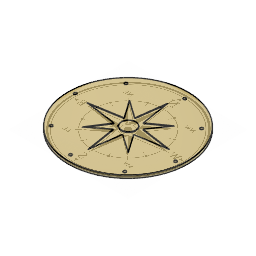
middle lid (Autodesk Fusion 360 design; units mm, degrees)
part number: 2026-06-30-11-55-46-724
Autodesk Fusion 360 part; units mm, degrees
sketch "Sketch1" plane through (0, 0, 0) normal (0, 1, 0) x (1, 0, 0)
  circle A0 centre (0, 0) radius 51
  dimension "d4" = 102
  constraint coincident A0.centre origin
  measures "d4" diameter of A0
sketch "Sketch2" plane through (0, 0, 0) normal (0, 1, 0) x (1, 0, 0)
  circle A0 centre (3.734, 44.6441) radius 1.2
  circle A1 centre (33.0064, 29.8467) radius 1.2
  circle A2 centre (46.1628, -5.5898) radius 1.2
  circle A3 centre (31.9934, -34.8384) radius 1.2
  circle A4 centre (-3.5224, -45.5641) radius 1.2
  circle A5 centre (-33.23, -32.3841) radius 1.2
  circle A6 centre (-46.7, 1.7546) radius 1.2
  circle A7 centre (-32.6391, 30.8334) radius 1.2
  dimension "d2" = 2.4
  dimension "d3" = 44.8
  dimension "d5" = 2.4
  dimension "d6" = 44.5
  dimension "d7" = 32.8
  dimension "d8" = 2.4
  dimension "d9" = 46.5
  dimension "d11" = 37.8
  dimension "d12" = 2.4
  dimension "d13" = 47.3
  dimension "d14" = 32.5
  dimension "d15" = 2.4
  dimension "d16" = 45.7
  dimension "d17" = 37.1
  dimension "d18" = 2.4
  dimension "d19" = 46.4
  dimension "d20" = 32.5
  dimension "d21" = 2.4
  dimension "d22" = 46.7
  dimension "d23" = 36.7
  dimension "d24" = 2.4
  dimension "d25" = 44.9
  dimension "d26" = 32.3
  dimension "d27" = 38.9067
  measures "d2" diameter of A0
  measures "d3" distance of A0.centre origin
  measures "d5" diameter of A1
  measures "d6" distance of origin A1.centre
  measures "d7" distance of A0.centre A1.centre
  measures "d8" diameter of A2
  measures "d9" distance of origin A2.centre
  measures "d11" distance of A1.centre A2.centre
  measures "d12" diameter of A3
  measures "d13" distance of origin A3.centre
  measures "d14" distance of A2.centre A3.centre
  measures "d15" diameter of A4
  measures "d16" distance of origin A4.centre
  measures "d17" distance of A3.centre A4.centre
  measures "d18" diameter of A5
  measures "d19" distance of origin A5.centre
  measures "d20" distance of A4.centre A5.centre
  measures "d21" diameter of A6
  measures "d22" horizontal distance of origin A6.centre
  measures "d23" distance of A5.centre A6.centre
  measures "d24" diameter of A7
  measures "d25" distance of origin A7.centre
  measures "d26" distance of A6.centre A7.centre
  measures "d27" distance of A0.centre A7.centre
extrude "Extrude1" add sketch "Sketch1" along normal blind 1.5
extrude "Extrude2" cut sketch "Sketch2" along normal blind 1.5
sketch "Sketch3" plane through (0, 0, 0) normal (0, 1, 0) x (1, 0, 0)
  circle A0 centre (0, 0.5) radius 6.1239
  line L0 (-3.8199, 5.2866) -> (0, 34)
  line L1 (0, 34) -> (4.8165, 4.282)
  line L2 (4.2751, 4.8848) -> (34.5625, 0.5686)
  line L3 (34.5625, 0.5686) -> (4.2751, -4.3402)
  line L4 (4.2751, -4.3402) -> (0, -34)
  line L5 (0, -34) -> (-5.024, -3.0016)
  line L6 (-3.9847, -4.1502) -> (-35, 0)
  line L7 (-35, 0) -> (-3.8199, 5.2866)
  line L8 (-8.4228, -3.5564) -> (-19, -20)
  line L9 (-19, -20) -> (-4.1619, -8.3209)
  line L10 (3.7013, -8.3209) -> (19.4188, -19.1701)
  line L11 (19.4188, -19.1701) -> (8.5353, -3.6497)
  line L12 (8.5353, 4.2777) -> (19.4188, 19.9901)
  line L13 (19.4188, 19.9901) -> (4.0404, 9.0706)
  line L14 (-3.3165, 9.0706) -> (-18.7508, 19.9901)
  line L15 (-18.7508, 19.9901) -> (-7.8613, 4.6013)
  constraint coincident A0 L0.start
  constraint coincident A0 L1.end
  constraint coincident A0 L2.start
  constraint perpendicular L1 L3
  constraint coincident A0 L5.end
  constraint perpendicular L3 L5
  constraint coincident A0 L6.start
  constraint coincident L6 L8.start
  constraint coincident L5 L9.end
  constraint coincident L4 L10.start
  constraint coincident L3 L11.end
  constraint coincident L2 L12.start
  constraint coincident L1 L13.end
  constraint coincident L0 L14.start
  constraint coincident L7 L15.end
extrude "Extrude3" cut sketch "Sketch3" along normal blind 1
extrude "Extrude4" add 1 faces at (-0.9503, 1.5, -4.8846) along direction (0, 1, 0) blind 1
emboss "Emboss1" depth -0.5 profiles "Sketch3" section 1 contours A0 L1 L2 L3 L4 L5 L6 | A0 L0 L1 L2 | L1 L2 L12 L13 | A0 L5 L6 L7 | L5 L6 L8 L9 | L0 L7 L14 L15 | L3 L4 L10 L11 onto face at (-0.9503, 2.5, -4.8846)
extrude "Extrude5" add 1 faces at (-17.0947, 1, -0.3483) along direction (0, -1, 0) blind 1
